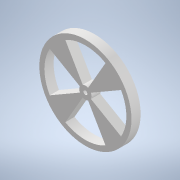
# Autodesk Inventor part: Pieza43
Saved by Autodesk Inventor 2022.2 (Build 262287000, 287)
## iProperties
Created: 2022-02-11
Part Number: Pieza43
Material: Genérico
Document SubType Name: Modeling
Designer: USUARIO
Density: 1 g/cm^3
Appearance: Valor por defecto
Author: USUARIO
Autodesk Inventor part; units mm, degrees
ref_plane "YZ Plane" through (0, 0, 0) normal (1, 0, 0) x (0, 1, 0)
ref_plane "XZ Plane" through (0, 0, 0) normal (0, 1, 0) x (-1, 0, 0)
ref_plane "XY Plane" through (0, 0, 0) normal (0, 0, 1) x (1, 0, 0)
sketch "Boceto1" plane through (0, 0, 0) normal (0, 0, 1) x (1, 0, 0)
  circle A0 centre (0, 0) radius 9.525
  circle A1 centre (0, 0) radius 225
  arc A2 (26.9272, -13.2259) -> (26.9272, 13.2259) centre (0, 0) ccw
  arc A3 (174.2011, -98.2546) -> (174.2011, 98.2546) centre (0, 0) ccw
  line L0 (26.9272, 13.2259) -> (174.2011, 98.2546)
  line L1 (26.9272, -13.2259) -> (174.2011, -98.2546)
  line L2 (13.2259, -26.9272) -> (98.2546, -174.2011)
  arc A4 (-98.2546, -174.2011) -> (98.2546, -174.2011) centre (0, 0) ccw
  line L3 (-13.2259, -26.9272) -> (-98.2546, -174.2011)
  arc A5 (-13.2259, -26.9272) -> (13.2259, -26.9272) centre (0, 0) ccw
  line L4 (-26.9272, -13.2259) -> (-174.2011, -98.2546)
  arc A6 (-174.2011, 98.2546) -> (-174.2011, -98.2546) centre (0, 0) ccw
  line L5 (-26.9272, 13.2259) -> (-174.2011, 98.2546)
  arc A7 (-26.9272, 13.2259) -> (-26.9272, -13.2259) centre (0, 0) ccw
  line L6 (-13.2259, 26.9272) -> (-98.2546, 174.2011)
  arc A8 (98.2546, 174.2011) -> (-98.2546, 174.2011) centre (0, 0) ccw
  line L7 (13.2259, 26.9272) -> (98.2546, 174.2011)
  arc A9 (13.2259, 26.9272) -> (-13.2259, 26.9272) centre (0, 0) ccw
  dimension "d2" = 450
  dimension "d3" = 60
  dimension "d4" = 400
  dimension "d11" = 360
  constraints: 16 end point, 16 point on circle, 10 centre point, 9 coincident, 43 other
  measures "d2" diameter of A1
  measures "d3" diameter of A2
  measures "d4" diameter of A3
extrude "Extrusión1" add sketch "Boceto1" along normal blind 45
